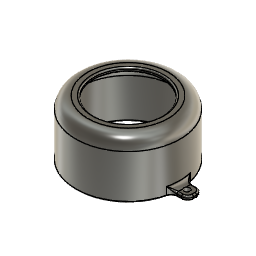
sheath (Autodesk Fusion 360 design; units mm, degrees)
Autodesk Fusion 360 part; units mm, degrees
sketch "Sketch1" plane through (0, 0, 0) normal (0, 0, 1) x (1, 0, 0)
  circle A0 centre (0, 0) radius 35
  circle A1 centre (0, 0) radius 32
  dimension "d1" = 70
  dimension "d2" = -3
  constraint coincident A0.centre A1.centre
  measures "d1" diameter of A0
extrude "Extrude1" add sketch "Sketch1" along normal blind 38
sketch "Sketch2" plane through (0, 0, 38) normal (0, 0, 1) x (-1, 0, 0)
  circle A0 centre (0, 0) radius 32
  circle A1 centre (0, 0) radius 35
  circle A2 centre (0, 0) radius 35
  circle A3 centre (0, 0) radius 23
  circle A4 centre (0, 0) radius 32
  dimension "d5" = 46
  constraint coincident A0.centre A1.centre
  constraint concentric A2 A4
  measures "d5" diameter of A3
extrude "Extrude2" add sketch "Sketch2" against normal blind 3 contours A0 A4
fillet "Fillet1" radius 8 1 edges at (-29.8345, -11.5717, 35)
fillet "Fillet2" radius 8 1 edges at (-32.6315, -12.6565, 38)
sketch "Sketch3" plane through (0, 0, 0) normal (0, 0, -1) x (1, 0, 0)
  circle A0 centre (0, 0) radius 32
  circle A1 centre (0, 0) radius 35
  line L0 (0, 0) -> (39.625, 0)
  circle A2 centre (39.625, 0) radius 2
  line L1 (35, 0) -> (45, 0)
  line L2 (45, 0) -> (45, -5)
  line L3 (45, -5) -> (34.641, -5)
  line L4 (45, 0) -> (45, 5)
  line L5 (45, 5) -> (34.641, 5)
  line L6 (0, 0) -> (0, -10)
  circle A3 centre (-39.625, 0) radius 2
  line L7 (-45, -5) -> (-34.641, -5)
  line L8 (-45, 0) -> (-45, -5)
  line L9 (-45, 0) -> (-45, 5)
  line L10 (-45, 5) -> (-34.641, 5)
  dimension "d12" = 39.625
  dimension "d13" = 4
  dimension "d14" = 10
  dimension "d15" = 5
  dimension "d16" = 5
  constraint coincident A0.centre A1.centre
  constraint horizontal L0
  constraint coincident L0.end A2.centre
  constraint coincident L0 L1.start
  constraint coincident A1 L1.start
  constraint parallel L0 L1
  constraint perpendicular L1 L2
  constraint coincident A1 L3.end
  constraint perpendicular L2 L3
  constraint perpendicular L1 L4
  constraint coincident A1 L5.end
  constraint perpendicular L4 L5
  constraint perpendicular L0 L6
  constraint symmetric A2 L6 A3
  constraint symmetric L1.end L6 L8.start
  constraint symmetric L2.end L6 L7.start
  constraint symmetric L3.end L6 L7.end
  constraint symmetric L4.end L6 L9.end
  constraint symmetric L5.end L6 L10.end
  measures "d12" distance of A0.centre L0.end
  measures "d13" diameter of A2
  measures "d14" distance of L1.start L1.end
  measures "d15" distance of L1.end L2.end
  measures "d16" distance of L1.end L4.end
extrude "Extrude3" add sketch "Sketch3" against normal blind 3 contours A1 L0 A2 L1 L2 L3 | A1 L0 A2 L1 L4 L5 | A1 L7 L8 L9 L10
fillet "Fillet3" radius 4 8 edges at (45, 5, 1.5) (45, -5, 1.5) (34.641, 5, 1.5) (34.641, -5, 1.5) (-34.641, -5, 1.5) (-45, -5, 1.5) (-45, 5, 1.5) (-34.641, 5, 1.5)
fillet "Fillet4" radius 3 2 edges at (-35, 0, 3) (35, 0, 3)
fillet "Fillet5" radius 1 37 edges at (35.197, 6.0956, 4.0491) (37.8077, 5.0024, 3) (39.4737, 5, 3) (43.8284, 3.8284, 3) (45, 0, 3) (43.8284, -3.8284, 3) (39.4737, -5, 3) (37.8077, -5.0024, 3) (35.1967, -6.0958, 4.0493) (35.4666, 5.8621, 0) (0, 35, 0) (-35.4666, 5.8621, 0) (-39.4737, 5, 0) (-43.8284, 3.8284, 0) (-45, 0, 0) (-43.8284, -3.8284, 0) (-39.4737, -5, 0) (-35.4666, -5.8621, 0) (0, -35, 0) (35.4666, -5.8621, 0) (39.4737, -5, 0) (43.8284, -3.8284, 0) (45, 0, 0) (43.8284, 3.8284, 0) (39.4737, 5, 0) (-35.197, -6.0956, 4.0491) (-37.8077, -5.0024, 3) (-39.4737, -5, 3) (-43.8284, -3.8284, 3) (-45, 0, 3) (-43.8284, 3.8284, 3) (-39.4737, 5, 3) (-37.8077, 5.0024, 3) (-35.1967, 6.0958, 4.0493) (-29.8345, 11.5717, 0) (21.4435, -8.3172, 38) (21.4435, 8.3172, 35)
